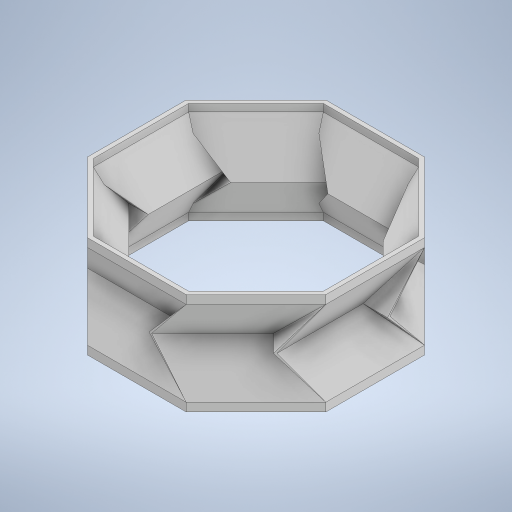
# Autodesk Inventor part: OV-PAM_half_scale2_1F
Saved by Autodesk Inventor 2024 (Build 280153000, 153)
## iProperties
Created: 2023-06-16
Part Number: OV-PAM_half_scale2_1F
Material: 일반
Document SubType Name: Modeling
Designer: jsw
Density: 1 g/cm^3
Appearance: 기본값
Author: jsw
Autodesk Inventor part; units mm, degrees
ref_plane "YZ Plane" through (0, 0, 0) normal (1, 0, 0) x (0, 1, 0)
ref_plane "XZ Plane" through (0, 0, 0) normal (0, 1, 0) x (-1, 0, 0)
ref_plane "XY Plane" through (0, 0, 0) normal (0, 0, 1) x (1, 0, 0)
sketch "스케치1" plane through (0, 0, 0) normal (0, 1, 0) x (-1, 0, 0)
  line L0 (-16.2959, 6.75) -> (-6.75, 16.2959)
  line L1 (-6.75, 16.2959) -> (6.75, 16.2959)
  line L2 (6.75, 16.2959) -> (16.2959, 6.75)
  line L3 (16.2959, 6.75) -> (16.2959, -6.75)
  line L4 (16.2959, -6.75) -> (6.75, -16.2959)
  line L5 (6.75, -16.2959) -> (-6.75, -16.2959)
  line L6 (-6.75, -16.2959) -> (-16.2959, -6.75)
  line L7 (-16.2959, -6.75) -> (-16.2959, 6.75)
  line L8 (-6.9985, 16.8959) -> (6.9985, 16.8959)
  line L9 (6.9985, 16.8959) -> (16.8959, 6.9985)
  line L10 (16.8959, 6.9985) -> (16.8959, -6.9985)
  line L11 (16.8959, -6.9985) -> (6.9985, -16.8959)
  line L12 (6.9985, -16.8959) -> (-6.9985, -16.8959)
  line L13 (-6.9985, -16.8959) -> (-16.8959, -6.9985)
  line L14 (-16.8959, -6.9985) -> (-16.8959, 6.9985)
  line L15 (-16.8959, 6.9985) -> (-6.9985, 16.8959)
  point P0 (0, 0)
  point P1 (0, 0)
  point P2 (0, 0)
  dimension "d0" = 13.5
  dimension "d2" = 0.6
  constraints: 32 end point, 2 coincident, 2 horizontal, 34 other
  measures "d0" distance of L0.end L1.end
  measures "d2" distance between parallel lines of L10 L3
extrude "돌출2" add sketch "스케치1" along normal blind 6 contours L0 L1 L2 L3 L4 L5 L6 L7 | L8 L9 L10 L11 L12 L13 L14 L15
ref_plane "작업 평면2" through (16.8959, 0, 6.9985) normal (-0.8660254, -0.5, 0) x (0, 0, -1)
sketch "스케치3" plane through (16.8959, 0, 6.9985) normal (1, 0, 0) x (0, 0, -1)
  line L0 (0, 0) -> (0, 6) projected
  line L1 (0, 6) -> (13.9971, 6) projected
  line L2 (0, 0) -> (13.9971, 0)
  line L3 (13.9971, 0) -> (13.9971, 6)
  line L4 (13.9971, 6) -> (0, 6)
  line L5 (0, 6) -> (0, 0)
  line L6 (0, 6) -> (-3.6524, 6)
  line L7 (-9.8974, 6) -> (0, 6) projected
  line L8 (0, 0) -> (-3.6524, 6)
  line L9 (13.9971, 6) -> (6.9985, 6)
  line L10 (8.7485, 6) -> (13.9971, 0)
  point P0 (6.9985, 0)
  point P1 (6.9985, 6)
  dimension "d17" = 121.33
  dimension "d54" = 1.75
  constraints: 16 end point, 6 midpoint, 2 parallel, 2 point on line, 1 horizontal, 1 perpendicular
  measures "d17" angle of L8 L2
  measures "d54" distance of L9.end L10.start
extrude "돌출4" cut sketch "스케치3" against normal up to surface contours L8 L6 L0 | L0 L1 L10 L2 surface through (16.8959, 0, 6.9985) normal (-0.8660254, -0.5, 0)
pattern_circular "원형 패턴1" count 8 over 360 about axis through (0, -10, 0) along (0, 1, 0) of "돌출4"
mirror "미러5" about plane through (0, 6, 0) normal (0, 1, 0) of "돌출2", "돌출4", "원형 패턴1"
ref_plane "작업 평면7" through (0, 6, 0) normal (0, -1, 0) x (1, 0, 0)
sketch "스케치14" plane through (-6.9985, 12, -16.8959) normal (0, 1, 0) x (1, 0, 0)
  line L0 (23.8945, -23.8945) -> (23.8945, -9.8974) projected
  line L1 (23.8945, -9.8974) -> (13.9971, 0) projected
  line L2 (13.9971, 0) -> (0, 0) projected
  line L3 (0, 0) -> (-9.8974, -9.8974) projected
  line L4 (-9.8974, -9.8974) -> (-9.8974, -23.8945) projected
  line L5 (-9.8974, -23.8945) -> (0, -33.7919) projected
  line L6 (0, -33.7919) -> (13.9971, -33.7919) projected
  line L7 (13.9971, -33.7919) -> (23.8945, -23.8945) projected
  point P0 (6.9985, -16.8959)
extrude "돌출11" add sketch "스케치14" along normal blind 1.2
mirror "미러9" about plane through (0, 6, 0) normal (0, -1, 0) of "돌출11"
shell "쉘10" thickness 0.6 removed faces 2 at (2.3328, 13.2, -0.9663) at (2.3328, -1.2, -0.9663)
